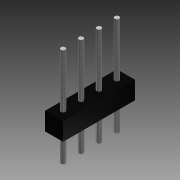
# Autodesk Inventor part: 2mm4PosHeader
Saved by Autodesk Inventor 2014 (Build 180170000, 170)
## iProperties
Created: 2015-11-06
Part Number: 2mm4PosHeader
Material: Generic
Document SubType Name: Modeling
Designer: Owner
Density: 1 g/cm^3
Appearance: Smooth - Black
Author: Owner
Autodesk Inventor part; units mm, degrees
ref_plane "YZ Plane" through (0, 0, 0) normal (1, 0, 0) x (0, 1, 0)
ref_plane "XZ Plane" through (0, 0, 0) normal (0, 1, 0) x (-1, 0, 0)
ref_plane "XY Plane" through (0, 0, 0) normal (0, 0, 1) x (1, 0, 0)
sketch "Sketch1" plane through (0, 0, 0) normal (0, 1, 0) x (-1, 0, 0)
  line L0 (-0.7674, 1.6667) -> (1.2326, 1.6667)
  line L1 (1.2326, 1.6667) -> (1.2326, -6.3333)
  line L2 (1.2326, -6.3333) -> (-0.7674, -6.3333)
  line L3 (-0.7674, -6.3333) -> (-0.7674, 1.6667)
  point P0 (0, 0)
  dimension "d0" = 2
  dimension "d1" = 8
  constraints: 8 end point, 2 parallel, 1 horizontal, 1 perpendicular
  measures "d0" distance of L0.start L0.end
  measures "d1" distance of L0.end L1.end
extrude "Extrusion1" add sketch "Sketch1" along normal blind 2
sketch "Sketch2" plane through (0, 2, 0) normal (0, 1, 0) x (1, 0, 0)
  line L0 (0.7674, 6.3333) -> (-1.2326, 6.3333) projected
  circle A0 centre (-0.2326, 5.3333) radius 0.25
  point P0 (0, 0)
  dimension "d4" = 1
  dimension "d5" = 0.5
  constraints: 1 centre point
  measures "d4" distance from line of L0 A0.centre
  measures "d5" diameter of A0
extrude "Extrusion2" add sketch "Sketch2" along normal blind 6 and the other way blind 5
pattern_linear "Rectangular Pattern1" count 4 spacing 2 along (0, 0, 1) of "Extrusion2"
body "Solid1"
